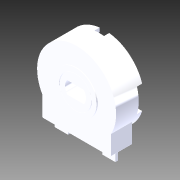
# Autodesk Inventor part: 276-2216.html
Saved by Autodesk Inventor 2013 (Build 170138000, 138)
## iProperties
Category: Sensors
Company: Autodesk Inc.
Created: 2012-04-08
Part Number: 276-2216.html
Document SubType Name: Modeling
Designer: Autodesk Inc.
Density: 1.42 g/cm^3
Material: Acetal Resin, White
Catalog Web Link: http://www.vexrobotics.com/products/accessories/sensors/276-2216.html
Vendor: VEX
Mass: 1.1586 g
Surface Area: 7.56442 cm^2
Volume: 0.815914 cm^3
Author: Autodesk Inc.
Autodesk Inventor part; units mm, degrees
ref_plane "YZ Plane" through (0, 0, 0) normal (1, 0, 0) x (0, 1, 0)
ref_plane "XZ Plane" through (0, 0, 0) normal (0, 1, 0) x (-1, 0, 0)
ref_plane "XY Plane" through (0, 0, 0) normal (0, 0, 1) x (1, 0, 0)
sketch "Sketch1" plane through (0, 0, 0) normal (0, 0, 1) x (1, 0, 0)
  arc A0 (6.5, -3.7417) -> (-6.5, -3.7417) centre (0, 0) ccw
  line L0 (-6.5, -7.3) -> (-6.5, -3.7417)
  arc A1 (-6.5, -7.3) -> (-6.3, -7.5) centre (-6.3, -7.3) ccw
  line L1 (6.3, -7.5) -> (-6.3, -7.5)
  arc A2 (6.3, -7.5) -> (6.5, -7.3) centre (6.3, -7.3) ccw
  line L2 (6.5, -3.7417) -> (6.5, -7.3)
  circle A3 centre (0, 0) radius 4
  constraints: 6 end point, 6 point on circle, 4 centre point
extrude "Extrusion1" add sketch "Sketch1" against normal blind 4.2926 contours L2 A2 L1 A1 L0 A0 | A3
sketch "Sketch2" plane through (0, 0, -4.2926) normal (0, 0, -1) x (-1, 0, 0)
  arc A0 (0.9, -6.6897) -> (6.364, -2.25) centre (0, 0) ccw
  line L0 (6.364, -2.25) -> (7.1545, -2.25)
  arc A1 (7.1545, -2.25) -> (7.1545, 2.25) centre (0, 0) ccw
  line L1 (7.1545, 2.25) -> (6.364, 2.25)
  arc A2 (6.364, 2.25) -> (0.9, 6.6897) centre (0, 0) ccw
  line L2 (0.9, 6.6897) -> (0.9, 7.4458)
  arc A3 (0.9, 7.4458) -> (-0.9, 7.4458) centre (0, 0) ccw
  line L3 (-0.9, 7.4458) -> (-0.9, 6.6897)
  arc A4 (-0.9, 6.6897) -> (-6.364, 2.25) centre (0, 0) ccw
  line L4 (-6.364, 2.25) -> (-7.1545, 2.25)
  arc A5 (-7.1545, 2.25) -> (-7.1545, -2.25) centre (0, 0) ccw
  line L5 (-7.1545, -2.25) -> (-6.364, -2.25)
  arc A6 (-6.364, -2.25) -> (-0.9, -6.6897) centre (0, 0) ccw
  line L6 (-0.9, -6.6897) -> (-0.9, -7.4458)
  arc A7 (-1.25, -7.3951) -> (-0.9, -7.4458) centre (0, 0) ccw
  arc A8 (0.9, -7.4458) -> (1.25, -7.3951) centre (0, 0) ccw
  line L7 (0.9, -7.4458) -> (0.9, -6.6897)
  arc A9 (1.6, -1.2) -> (1.6, 1.2) centre (0, 0) ccw
  line L8 (1.6, -1.2) -> (-1.6, -1.2)
  arc A10 (-1.6, 1.2) -> (-1.6, -1.2) centre (0, 0) ccw
  line L9 (1.6, 1.2) -> (-1.6, 1.2)
  arc A11 (-1.25, -7.3951) -> (-0.9, -7.4458) centre (0, 0) ccw
  arc A12 (-7.1545, -2.25) -> (-1.25, -7.3951) centre (0, 0) ccw
  arc A13 (-7.1545, 2.25) -> (-7.1545, -2.25) centre (0, 0) ccw
  arc A14 (-0.9, 7.4458) -> (-7.1545, 2.25) centre (0, 0) ccw
  arc A15 (0.9, 7.4458) -> (-0.9, 7.4458) centre (0, 0) ccw
  arc A16 (7.1545, 2.25) -> (0.9, 7.4458) centre (0, 0) ccw
  arc A17 (7.1545, -2.25) -> (7.1545, 2.25) centre (0, 0) ccw
  arc A18 (1.25, -7.3951) -> (7.1545, -2.25) centre (0, 0) ccw
  line L10 (-0.9, -6.6897) -> (-0.9, -7.4458)
  arc A19 (-6.364, -2.25) -> (-0.9, -6.6897) centre (0, 0) ccw
  line L11 (-7.1545, -2.25) -> (-6.364, -2.25)
  line L12 (-6.364, 2.25) -> (-7.1545, 2.25)
  arc A20 (-0.9, 6.6897) -> (-6.364, 2.25) centre (0, 0) ccw
  line L13 (-0.9, 7.4458) -> (-0.9, 6.6897)
  line L14 (0.9, 6.6897) -> (0.9, 7.4458)
  arc A21 (6.364, 2.25) -> (0.9, 6.6897) centre (0, 0) ccw
  line L15 (7.1545, 2.25) -> (6.364, 2.25)
  line L16 (6.364, -2.25) -> (7.1545, -2.25)
  arc A22 (0.9, -6.6897) -> (6.364, -2.25) centre (0, 0) ccw
  line L17 (0.9, -7.4458) -> (0.9, -6.6897)
  arc A23 (0.9, -7.4458) -> (1.25, -7.3951) centre (0, 0) ccw
  arc A24 (1.6, -1.2) -> (1.6, 1.2) centre (0, 0) ccw
  line L18 (1.6, 1.2) -> (-1.6, 1.2)
  arc A25 (-1.6, 1.2) -> (-1.6, -1.2) centre (0, 0) ccw
  line L19 (-1.6, -1.2) -> (1.6, -1.2)
  constraints: 52 point on circle, 40 end point, 26 centre point
extrude "Extrusion2" add sketch "Sketch2" along normal blind 0.9906 contours L5 A6 L6 A7 A12 | L3 A4 L4 A14 | L1 A2 L2 A16 | A0 L0 A18 A8 L7
extrude "Extrusion3" cut sketch "Sketch2" against normal up to next contours L8 A10 L9 A9
sketch "Sketch3" plane through (0, 0, 0) normal (0, 0, 1) x (1, 0, 0)
  arc A0 (1.6, -1.2) -> (1.6, 1.2) centre (0, 0) ccw projected
  line L0 (1.6, -1.2) -> (-1.6, -1.2) projected
  arc A1 (-1.6, 1.2) -> (-1.6, -1.2) centre (0, 0) ccw projected
  line L1 (-1.6, 1.2) -> (1.6, 1.2) projected
  arc A2 (6.5, -3.7417) -> (-6.5, -3.7417) centre (0, 0) ccw
  line L2 (-6.5, -7.3) -> (-6.5, -3.7417)
  arc A3 (-6.5, -7.3) -> (-6.3, -7.5) centre (-6.3, -7.3) ccw
  line L3 (6.3, -7.5) -> (-6.3, -7.5)
  arc A4 (6.3, -7.5) -> (6.5, -7.3) centre (6.3, -7.3) ccw
  line L4 (6.5, -3.7417) -> (6.5, -7.3)
  circle A5 centre (0, 0) radius 4
  circle A6 centre (0, 0) radius 4
  circle A7 centre (0, 0) radius 3.075
  arc A8 (6.5, -3.7417) -> (-6.5, -3.7417) centre (0, 0) ccw
  line L5 (-6.5, -7.3) -> (-6.5, -3.7417)
  arc A9 (-6.5, -7.3) -> (-6.3, -7.5) centre (-6.3, -7.3) ccw
  line L6 (6.3, -7.5) -> (-6.3, -7.5)
  arc A10 (6.3, -7.5) -> (6.5, -7.3) centre (6.3, -7.3) ccw
  line L7 (6.5, -3.7417) -> (6.5, -7.3)
  circle A11 centre (0, 0) radius 4
  circle A12 centre (0, 0) radius 4
  circle A13 centre (0, 0) radius 3.075
  circle A14 centre (0, 0) radius 3
  line L8 (1.6, -1.2) -> (-1.6, -1.2)
  arc A15 (-1.6, 1.2) -> (-1.6, -1.2) centre (0, 0) ccw
  line L9 (-1.6, 1.2) -> (1.6, 1.2)
  arc A16 (1.6, -1.2) -> (1.6, 1.2) centre (0, 0) ccw
  constraints: 16 end point, 16 point on circle, 15 centre point
extrude "Extrusion4" add sketch "Sketch3" along normal blind 0.2032 contours A5 | A14
sketch "Sketch5" plane through (0, 0, -4.2926) normal (0, 0, -1) x (-1, 0, 0)
  arc A0 (-6.5, -3.7417) -> (-0.9, -7.4458) centre (0, 0) ccw projected
  line L0 (-6.5, -7.3) -> (-6.5, -3.7417) projected
  arc A1 (-6.5, -7.3) -> (-6.3, -7.5) centre (-6.3, -7.3) ccw projected
  line L1 (6.3, -7.5) -> (-6.3, -7.5) projected
  line L2 (6.5, -3.7417) -> (6.5, -7.3) projected
  arc A2 (0.9, -7.4458) -> (6.5, -3.7417) centre (0, 0) ccw projected
  arc A3 (-6.5, -3.7417) -> (0, -7.5) centre (0, 0) ccw
  line L3 (-6.5, -3.7417) -> (-6.5, -7.2968)
  line L4 (-6.2968, -7.5) -> (0, -7.5)
  line L5 (6.5, -7.2968) -> (6.5, -3.7417)
  arc A4 (-6.5, -7.2968) -> (-6.2968, -7.5) centre (-6.2968, -7.2968) ccw
  arc A5 (6.2968, -7.5) -> (6.5, -7.2968) centre (6.2968, -7.2968) ccw
  circle A6 centre (0, 0) radius 7.5
  point P0 (-6.5, -7.5)
  dimension "d8" = 0.2032
  constraints: 6 end point, 6 point on circle, 6 tangent, 3 centre point, 3 point on line, 1 coincident, 1 collinear, 1 equal radius, 1 midpoint, 1 perpendicular, 1 vertical alignment, 2 other
  measures "d8" radius of A4
extrude "Extrusion5" cut sketch "Sketch5" against normal blind 0.3048 contours A0 A3 L1 A1 L0
mirror "Mirror1" about plane through (0, 0, 0) normal (1, 0, 0) of "Extrusion5"
sketch "Sketch4" plane through (-6.3, -7.5, 0) normal (0, -1, 0) x (1, 0, 0)
  line L0 (0, -4.2926) -> (12.6, -4.2926) projected
  line L1 (5.05, -4) -> (0, -4)
  line L2 (5.05, -4.2926) -> (5.05, -3.8)
  line L3 (7.55, -3.8) -> (5.05, -3.8)
  line L4 (7.55, -4.2926) -> (7.55, -3.8)
  line L5 (12.6, -4) -> (7.55, -4)
  line L6 (12.6, -4) -> (12.6, 0)
  line L7 (12.6, 0) -> (0, 0)
  line L8 (0, -4) -> (0, 0)
  line L9 (3.05, -1.6) -> (0.55, -1.6)
  line L10 (3.05, -1.6) -> (3.05, -2.1)
  line L11 (3.05, -2.1) -> (0.55, -2.1)
  line L12 (0.55, -2.1) -> (0.55, -1.6)
  line L13 (12.05, -1.6) -> (9.55, -1.6)
  line L14 (12.05, -1.6) -> (12.05, -2.1)
  line L15 (12.05, -2.1) -> (9.55, -2.1)
  line L16 (9.55, -2.1) -> (9.55, -1.6)
  line L17 (7.55, -4.2926) -> (5.05, -4.2926)
  line L18 (7.55, -3.8) -> (5.05, -3.8)
  line L19 (5.05, -3.8) -> (5.05, -4.2926)
  line L20 (5.05, -4.2926) -> (7.55, -4.2926)
  line L21 (7.55, -4.2926) -> (7.55, -3.8)
  point P0 (6.3, 0)
  point P1 (6.3, 0)
  constraints: 42 end point, 5 point on line, 2 collinear, 2 parallel, 1 horizontal, 1 perpendicular, 1 vertical
extrude "Extrusion6" add sketch "Sketch4" along normal blind 2.0066 contours L10 L11 L12 L9 | L14 L15 L16 L13
extrude "Extrusion7" add sketch "Sketch4" along normal up to surface (2.0066 mm away) from surface at 0 contours L2 L3 L4 L0
body "Solid1"
